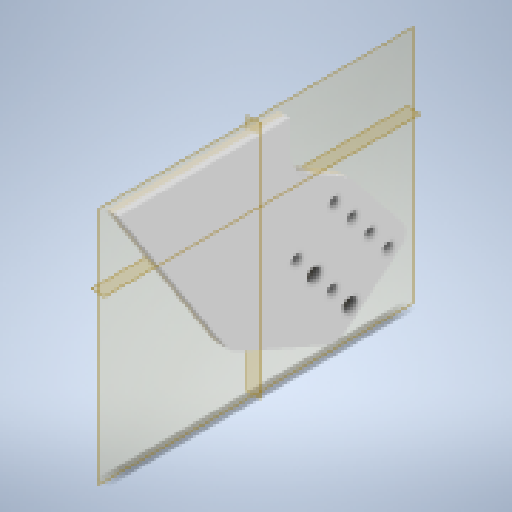
# Autodesk Inventor part: Крепление хвоста(2 часть)
Saved by Autodesk Inventor 2023.2 (Build 272271030, 271C)
## iProperties
Created: 2024-03-15
Part Number: Крепление хвоста(2 часть)
Material: Типовые
Document SubType Name: Modeling
Designer: I9232
Density: 1 g/cm^3
Appearance: По умолчанию
Author: I9232
Autodesk Inventor part; units mm, degrees
sketch "Эскиз1" plane through (0, 0, 0) normal (1, 0, 0) x (0, 1, 0)
  line L0 (20.1986, -10.0085) -> (5.0003, -9.9028)
  line L1 (-6.6279, -29.6225) -> (-22.2328, -42.1001)
  line L2 (-6.6279, -29.6225) -> (5.0003, -9.9028)
  line L3 (-36.5734, 10) -> (20.1986, 46.6306)
  line L4 (-36.5734, 10) -> (-52.1666, -25.2798)
  line L5 (-52.1666, -25.2798) -> (-31.9819, -50.0458)
  line L6 (-31.9819, -50.0458) -> (-22.2328, -42.1001)
  line L7 (20.1986, -10.0085) -> (20.1986, 46.6306)
  line L8 (-20.4694, -44.4074) -> (-42.8024, -17.0055)
  point P0 (0, 0)
  point P1 (-8.36, -30.6225)
  constraints: 16 end point, 1 parallel, 1 perpendicular, 1 vertical, 6 other
extrude "Выдавливание1" add sketch "Эскиз1" along normal mid plane 4
fillet "Сопряжение1" radius 10 3 edges at (0, -36.5734, 10) (0, -6.6279, -29.6225) (0, 5.0003, -9.9028)
fillet "Сопряжение2" radius 5 1 edges at (0, -22.2328, -42.1001)
sketch "Эскиз2" plane through (2, 0, 0) normal (1, 0, 0) x (0, 0, -1)
  circle A0 centre (36.0864, -25.5741) radius 1.5 projected
  circle A1 centre (24.2724, -11.0786) radius 1.5 projected
  circle A2 centre (11.8699, -21.1868) radius 1.5 projected
  circle A3 centre (23.6839, -35.6823) radius 1.5 projected
  point P0 (0, 0)
extrude "Выдавливание2" cut sketch "Эскиз2" against normal blind 4
sketch "Эскиз3" plane through (2, 0, 0) normal (1, 0, 0) x (0, 0, -1)
  circle A0 centre (30.1478, -18.2876) radius 1.5 projected
  line L0 (28.1052, -15.7813) -> (31.0975, -15.2977) projected
  line L1 (26.9561, -18.8034) -> (28.1052, -15.7813) projected
  line L2 (28.9987, -21.3096) -> (26.9561, -18.8034) projected
  line L3 (32.1904, -20.7938) -> (28.9987, -21.3096) projected
  line L4 (33.2678, -17.9606) -> (32.1904, -20.7938) projected
  line L5 (31.297, -15.2655) -> (33.3396, -17.7717) projected
  line L6 (33.2678, -17.9606) -> (33.3396, -17.7717) projected
  line L7 (31.297, -15.2655) -> (31.0975, -15.2977) projected
  circle A1 centre (17.7453, -28.3958) radius 1.5 projected
  circle A2 centre (17.7453, -28.3958) radius 2.25 projected
  point P0 (0, 0)
extrude "Выдавливание3" cut sketch "Эскиз3" against normal blind 4 contours A0 | A1 | A2
sketch "Эскиз4" plane through (2, 0, 0) normal (1, 0, 0) x (0, 0, -1)
  circle A0 centre (29.5593, -42.8913) radius 2.25 projected
  circle A1 centre (41.9619, -32.783) radius 2.25 projected
  circle A2 centre (41.9619, -32.783) radius 1.5 projected
  point P0 (0, 0)
extrude "Выдавливание4" cut sketch "Эскиз4" against normal blind 4 contours A0 | A2
fillet "Сопряжение3" radius 5 2 edges at (0, -52.1666, -25.2798) (0, -31.9819, -50.0458)
sketch "Эскиз5" plane through (-2, 20.1986, 46.6306) normal (0, 1, 0) x (1, 0, 0)
  line L0 (0, 56.5734) -> (4, 56.5734) projected
  line L1 (0, 0) -> (0, 56.639) projected
  line L2 (4, 56.5734) -> (0, 56.5734)
  line L3 (0, 56.5734) -> (0, 50.5734)
  line L4 (0, 50.5734) -> (4, 50.5734)
  line L5 (4, 50.5734) -> (4, 56.5734)
  line L6 (4, 56.639) -> (4, 0) projected
  line L7 (4, 40.5734) -> (0, 40.5734)
  line L8 (0, 40.5734) -> (0, 34.5734)
  line L9 (0, 34.5734) -> (4, 34.5734)
  line L10 (4, 34.5734) -> (4, 40.5734)
  line L11 (4, 0) -> (0, 0)
  line L12 (0, 0) -> (0, 6)
  line L13 (0, 6) -> (4, 6)
  line L14 (4, 6) -> (4, 0)
  line L15 (4, 16) -> (0, 16)
  line L16 (0, 16) -> (0, 22)
  line L17 (0, 22) -> (4, 22)
  line L18 (4, 22) -> (4, 16)
  point P0 (2, 46.6306)
  point P1 (4, 6)
  point P2 (4, 22)
  point P3 (0, 16)
  point P4 (4, 34.5734)
  point P5 (0, 40.5734)
  dimension "d13" = 6
  dimension "d14" = 6
  dimension "d15" = 10
  dimension "d16" = 6
  dimension "d17" = 10
  dimension "d18" = 6
  constraints: 32 end point, 8 parallel, 6 point on line, 4 horizontal, 4 perpendicular
  measures "d13" distance of L4.end L0.end
  measures "d14" distance of L9.end L7.start
  measures "d15" distance between parallel lines of L7 L4
  measures "d16" distance of L15.start L17.end
  measures "d17" distance between parallel lines of L13 L15
  measures "d18" distance of L6.end L13.end
extrude "Выдавливание5" add sketch "Эскиз5" along normal blind 4 contours L0 L5 L4 L1 | L7 L6 L9 L1 | L17 L6 L15 L1 | L13 L6 L11 L1
sketch "Эскиз6" plane through (2, 0, 0) normal (1, 0, 0) x (0, 0, -1)
  line L0 (-6.0571, 20.1986) -> (3.9429, 20.1986) projected
  line L1 (0.3929, 20.1986) -> (-2.5071, 20.1986)
  line L2 (-2.5071, 5.2986) -> (0.3929, 5.2986)
  line L3 (-1.0571, 5.2986) -> (-1.0571, 20.1986) construction
  line L4 (-3.8571, 10.2986) -> (-3.8571, 12.0986)
  line L5 (1.7429, 12.0986) -> (1.7429, 10.2986)
  line L6 (0.3929, 5.2986) -> (0.3929, 10.2986)
  line L7 (0.3929, 12.0986) -> (0.3929, 20.1986)
  line L8 (1.7429, 10.2986) -> (0.3929, 10.2986)
  line L9 (-2.5071, 10.2986) -> (-3.8571, 10.2986)
  line L10 (-3.8571, 12.0986) -> (-2.5071, 12.0986)
  line L11 (0.3929, 12.0986) -> (1.7429, 12.0986)
  line L12 (-2.5071, 20.1986) -> (-2.5071, 12.0986)
  line L13 (-2.5071, 10.2986) -> (-2.5071, 5.2986)
  line L14 (-34.1806, 20.1986) -> (-37.0806, 20.1986)
  line L15 (-37.0806, 10.8986) -> (-34.1806, 10.8986)
  line L16 (-35.6306, 10.8986) -> (-35.6306, 20.1986) construction
  line L17 (-38.4306, 13.8986) -> (-38.4306, 15.6986)
  line L18 (-32.8306, 15.6986) -> (-32.8306, 13.8986)
  line L19 (-34.1806, 10.8986) -> (-34.1806, 13.8986)
  line L20 (-34.1806, 15.6986) -> (-34.1806, 20.1986)
  line L21 (-32.8306, 13.8986) -> (-34.1806, 13.8986)
  line L22 (-37.0806, 13.8986) -> (-38.4306, 13.8986)
  line L23 (-38.4306, 15.6986) -> (-37.0806, 15.6986)
  line L24 (-34.1806, 15.6986) -> (-32.8306, 15.6986)
  line L25 (-37.0806, 20.1986) -> (-37.0806, 15.6986)
  line L26 (-37.0806, 13.8986) -> (-37.0806, 10.8986)
  line L27 (-30.6306, 20.1986) -> (-40.6306, 20.1986) projected
  point P0 (0, 0)
  point P1 (-3.8571, 11.1986)
  point P2 (1.7429, 11.1986)
  point P3 (-38.4306, 14.7986)
  point P4 (-32.8306, 14.7986)
  point P5 (-33.5056, 15.6986)
  point P6 (1.0679, 12.0986)
  dimension "d21" = 2.9
  dimension "d23" = 1.8
  dimension "d25" = 1.35
  dimension "d26" = 2.9
  dimension "d27" = 8.1
  dimension "d28" = 5
  dimension "d29" = 2.9
  dimension "d30" = 1.8
  dimension "d31" = 1.35
  dimension "d32" = 2.9
  dimension "d33" = 3
  dimension "d34" = 4.5
  dimension "d35" = 4.5
  dimension "d38" = 8.1
  constraints: 52 end point, 24 parallel, 12 midpoint, 8 perpendicular, 6 horizontal, 4 equal length, 1 point on line
  measures "d21" distance of L2.start L2.end
  measures "d23" distance of L5.start L5.end
  measures "d25" distance of L9.start L4.start
  measures "d26" distance between parallel lines of L12 L7
  measures "d27" distance between parallel lines of L0 L10
  measures "d28" distance of L9.start L2.start
  measures "d29" distance of L15.start L19.start
  measures "d30" distance of L18.start L21.start
  measures "d31" distance of L22.start L17.start
  measures "d32" distance between parallel lines of L25 L20
  measures "d33" distance of L22.start L15.start
  measures "d34" distance from line of L27 point (-33.506, 15.699)
  measures "d35" distance between parallel lines of L27 L23
  measures "d38" distance from line of L0 point (1.068, 12.099)
extrude "Выдавливание6" cut sketch "Эскиз6" against normal up to surface (4 mm away)
